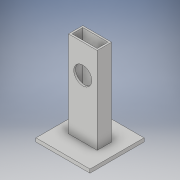
# Autodesk Inventor part: ThunderhexPost
Saved by Autodesk Inventor 2017 SP1 (Build 210196100, 196)
## iProperties
Created: 2016-08-08
Part Number: ThunderhexPost
Material: Generic
Document SubType Name: Modeling
Designer: steele
Density: 1 g/cm^3
Appearance: Default
Author: steele
Autodesk Inventor part; units mm, degrees
ref_plane "YZ Plane" through (0, 0, 0) normal (1, 0, 0) x (0, 1, 0)
ref_plane "XZ Plane" through (0, 0, 0) normal (0, 1, 0) x (-1, 0, 0)
ref_plane "XY Plane" through (0, 0, 0) normal (0, 0, 1) x (1, 0, 0)
sketch "Sketch1" plane through (0, 0, 0) normal (0, 1, 0) x (-1, 0, 0)
  line L0 (47.625, 47.625) -> (-47.625, 47.625)
  line L1 (-47.625, 47.625) -> (-47.625, -47.625)
  line L2 (-47.625, -47.625) -> (47.625, -47.625)
  line L3 (47.625, -47.625) -> (47.625, 47.625)
  line L4 (47.625, 47.625) -> (-47.625, -47.625) construction
  line L5 (-47.625, 47.625) -> (47.625, -47.625) construction
  point P0 (0, 0)
  dimension "d0" = 95.25
  constraints: 12 end point, 2 midpoint, 2 parallel, 2 perpendicular, 1 horizontal
  measures "d0" distance of L0.start L0.end
extrude "Extrusion1" add sketch "Sketch1" against normal blind 6.35
sketch "Sketch2" plane through (0, 0, 0) normal (0, 1, 0) x (1, 0, 0)
  line L0 (-25.4, -12.7) -> (25.4, -12.7)
  line L1 (25.4, -12.7) -> (25.4, 12.7)
  line L2 (25.4, 12.7) -> (-25.4, 12.7)
  line L3 (-25.4, 12.7) -> (-25.4, -12.7)
  line L4 (-25.4, -12.7) -> (25.4, 12.7) construction
  line L5 (25.4, -12.7) -> (-25.4, 12.7) construction
  line L6 (-22.225, -9.525) -> (22.225, -9.525)
  line L7 (22.225, -9.525) -> (22.225, 9.525)
  line L8 (22.225, 9.525) -> (-22.225, 9.525)
  line L9 (-22.225, 9.525) -> (-22.225, -9.525)
  line L10 (-22.225, -9.525) -> (22.225, 9.525) construction
  line L11 (22.225, -9.525) -> (-22.225, 9.525) construction
  point P0 (0, 0)
  dimension "d3" = 50.8
  dimension "d4" = 25.4
  dimension "d5" = 3.175
  dimension "d6" = 3.175
  constraints: 24 end point, 4 midpoint, 4 parallel, 2 horizontal, 2 perpendicular
  measures "d3" distance of L0.start L0.end
  measures "d4" distance of L2.end L0.start
  measures "d5" distance between parallel lines of L6 L0
  measures "d6" distance between parallel lines of L1 L7
extrude "Extrusion2" add sketch "Sketch2" along normal blind 152.4
sketch "Sketch3" plane through (-25.4, 0, 12.7) normal (0, 0, 1) x (1, 0, 0)
  line L0 (25.4, 0) -> (25.4, 152.4) construction
  line L1 (0, 152.4) -> (50.8, 152.4) construction
  line L2 (-22.225, 0) -> (73.025, 0) construction
  point P0 (25.4, 101.6)
  dimension "d9" = 101.6
  constraints: 2 end point, 1 midpoint, 1 point on line
  measures "d9" distance from line of point (25.4, 101.6) L2
hole "Hole1" at (0, 101.6, 12.7) direction (0, 0, -1) diameter 31.75 end up to face face through (-7.4083, 50.8, 9.525) facing (0, 0, -1)
sketch "Sketch4" plane through (25.4, 0, -12.7) normal (0, 0, -1) x (-1, 0, 0)
  line L0 (25.4, 0) -> (25.4, 152.4) construction
  line L1 (50.8, 152.4) -> (0, 152.4) construction
  circle A0 centre (25.4, 101.6) radius 15.875 projected
  constraints: 2 end point, 1 coincident, 1 midpoint
hole "Hole2" at (0, 101.6, -12.7) direction (0, 0, 1) diameter 13.7414 end up to face face through (7.4083, 50.8, -9.525) facing (0, 0, 1)
equation "\"d1\" = baseMaterialThickness"
equation "\"d5\" = postMaterialThickness"
equation "\"d6\" = postMaterialThickness"
equation "\"d10\" = flangeBearingHoleDiam"
equation "\"flangeBearingHoleDiam\" = 31.75"
equation "\"heightOfRod\" = 101.6"
equation "\"hightOfPost\" = 152.4"
equation "\"postMaterialThickness\" = 3.175"
equation "\"baseMaterialThickness\" = 6.35"
body "Solid1"
